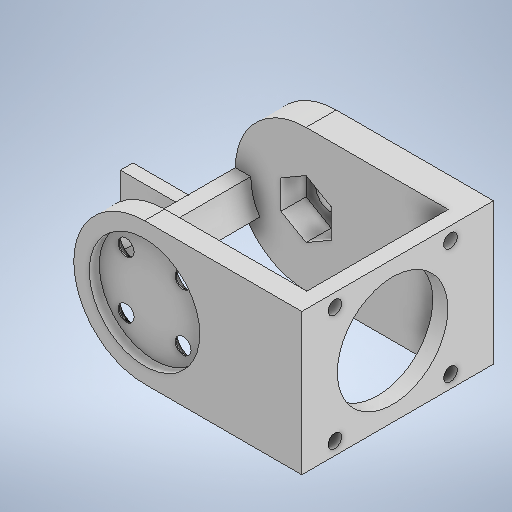
# Autodesk Inventor part: j6 motor mount v2
Saved by Autodesk Inventor 2025 (Build 290162000, 162)
## iProperties
Created: 2025-08-05
Part Number: j6 motor mount v2
Material: 一般
Document SubType Name: Modeling
Designer: gavin
Density: 1 g/cm^3
Appearance: 預設
Author: gavin
## iProperties of the stored document j6 motor mount v2_3D 列印.ipt
Created: 2025-08-05
Part Number: j6 motor mount v2_3D 列印
Material: 一般
Document SubType Name: Modeling
Designer: gavin
Density: 1 g/cm^3
Appearance: 預設
Author: gavin
Autodesk Inventor part; units mm, degrees
ref_plane "YZ Plane" through (0, 0, 0) normal (1, 0, 0) x (0, 1, 0)
ref_plane "XZ Plane" through (0, 0, 0) normal (0, 1, 0) x (-1, 0, 0)
ref_plane "XY Plane" through (0, 0, 0) normal (0, 0, 1) x (1, 0, 0)
sketch "草圖1" plane through (0, 0, 0) normal (1, 0, 0) x (0, 1, 0)
  line L0 (-14.075, 14.075) -> (14.075, 14.075)
  line L1 (14.075, 14.075) -> (14.075, -14.075)
  line L2 (14.075, -14.075) -> (-14.075, -14.075)
  line L3 (-14.075, -14.075) -> (-14.075, 14.075)
  line L4 (-14.075, 14.075) -> (14.075, -14.075) construction
  line L5 (14.075, 14.075) -> (-14.075, -14.075) construction
  line L6 (14.075, 14.075) -> (-14.075, 14.075)
  line L7 (-14.075, 14.075) -> (-14.075, 18.075)
  line L8 (-14.075, 18.075) -> (14.075, 18.075)
  line L9 (14.075, 18.075) -> (14.075, 14.075)
  circle A0 centre (0, 0) radius 11
  line L10 (-11.5, 11.5) -> (11.5, 11.5) construction
  line L11 (11.5, 11.5) -> (11.5, -11.5) construction
  line L12 (11.5, -11.5) -> (-11.5, -11.5) construction
  line L13 (-11.5, -11.5) -> (-11.5, 11.5) construction
  line L14 (-11.5, 11.5) -> (11.5, -11.5) construction
  line L15 (11.5, 11.5) -> (-11.5, -11.5) construction
  circle A1 centre (11.5, 11.5) radius 1.35
  circle A2 centre (-11.5, 11.5) radius 1.35
  circle A3 centre (-11.5, -11.5) radius 1.35
  circle A4 centre (11.5, -11.5) radius 1.35
  line L16 (14.075, -14.075) -> (-14.075, -14.075)
  line L17 (-14.075, -14.075) -> (-14.075, -20.075)
  line L18 (-14.075, -20.075) -> (14.075, -20.075)
  line L19 (14.075, -20.075) -> (14.075, -14.075)
  dimension "d0" = 28.15
  dimension "d1" = 28.15
  dimension "d2" = 4
  dimension "d3" = 22
  dimension "d4" = 23
  dimension "d5" = 23
  dimension "d6" = 2.7
  dimension "d9" = 360
  dimension "d11" = 6
  constraints: 40 end point, 8 parallel, 5 centre point, 4 horizontal, 4 midpoint, 4 perpendicular, 2 coincident, 9 other
  measures "d0" distance of L1.end L2.end
  measures "d1" distance of L0.end L1.end
  measures "d2" distance of L6.end L7.end
  measures "d3" diameter of A0
  measures "d4" distance of L11.end L12.end
  measures "d5" distance of L10.end L11.end
  measures "d6" diameter of A1
  measures "d11" distance of L17.end L16.end
extrude "擠出1" add sketch "草圖1" along normal blind 3
sketch "草圖2" plane through (0, 0, 0) normal (-1, 0, 0) x (0, 0, 1)
  line L0 (18.075, 14.075) -> (18.075, -14.075) projected
  line L1 (-20.075, 14.075) -> (18.075, 14.075) projected
  line L2 (-20.075, -14.075) -> (-20.075, 14.075) projected
  line L3 (18.075, -14.075) -> (-20.075, -14.075) projected
  circle A0 centre (0, 0) radius 11 projected
  circle A1 centre (11.5, 11.5) radius 1.35 projected
  circle A2 centre (11.5, -11.5) radius 1.35 projected
  circle A3 centre (-11.5, -11.5) radius 1.35 projected
  circle A4 centre (-11.5, 11.5) radius 1.35 projected
  line L4 (-14.075, 14.075) -> (-14.075, -14.075)
  line L5 (14.075, 14.075) -> (14.075, -14.075)
  dimension "d14" = 6
  dimension "d15" = 4
  constraints: 4 end point, 4 point on line, 2 vertical
  measures "d14" distance between parallel lines of L2 L4
  measures "d15" distance between parallel lines of L0 L5
extrude "擠出2" add sketch "草圖2" along normal blind 42.375 contours L0 L3 L5 L1 | L4 L3 L2 L1
sketch "草圖3" plane through (3, -14.075, 18.075) normal (0, 0, 1) x (1, 0, 0)
  line L0 (-45.375, 0) -> (0, 0) projected
  line L1 (0, 28.15) -> (0, 0) projected
  line L2 (0, 28.15) -> (-45.375, 28.15) projected
  line L3 (-45.375, 0) -> (-45.375, 28.15) projected
  circle A0 centre (-31.3, 14.075) radius 11
  line L4 (-45.375, 0) -> (-45.375, 28.15) projected
  circle A1 centre (-31.3, 14.075) radius 8 construction
  line L5 (-31.3, 14.075) -> (-23.5218, 21.8532) construction
  line L6 (-31.3, 14.075) -> (-20.3, 14.075) construction
  circle A2 centre (-25.6431, 19.7319) radius 1.6
  circle A3 centre (-36.9569, 19.7319) radius 1.6
  circle A4 centre (-36.9569, 8.4181) radius 1.6
  circle A5 centre (-25.6431, 8.4181) radius 1.6
  point P0 (-3, 14.075)
  dimension "d18" = 22
  dimension "d19" = 16
  dimension "d20" = 45
  dimension "d21" = 3.2
  dimension "d24" = 360
  dimension "d30" = 14.075
  dimension "d31" = 14.075
  constraints: 4 centre point, 4 end point, 1 coincident, 1 equal length, 1 horizontal, 1 horizontal alignment, 1 point on line, 15 other
  measures "d20" angle of L6 L5
  measures "d21" diameter of A2
  measures "d30" distance from line of L2 point (-31.3, 14.075)
  measures "d31" distance from line of L3 point (-31.3, 14.075)
extrude "擠出3" cut sketch "草圖3" against normal up to surface (4 mm away) contours A2 | A3 | A4 | A5
extrude "擠出4" cut sketch "草圖3" against normal blind 2 contours A0
fillet "圓角1" radius 14.075 4 edges at (-42.375, 14.075, 16.075) (-42.375, 14.075, -17.075) (-42.375, -14.075, 16.075) (-42.375, -14.075, -17.075)
sketch "草圖4" plane through (0, -14.075, -14.075) normal (0, 0, 1) x (1, 0, 0)
  circle A0 centre (-28.3, 14.075) radius 11 projected
  line L0 (-28.3, 8.3015) -> (-33.3, 11.1882)
  line L1 (-33.3, 11.1882) -> (-33.3, 16.9618)
  line L2 (-33.3, 16.9618) -> (-28.3, 19.8485)
  line L3 (-28.3, 19.8485) -> (-23.3, 16.9618)
  line L4 (-23.3, 16.9618) -> (-23.3, 11.1882)
  line L5 (-23.3, 11.1882) -> (-28.3, 8.3015)
  point P0 (0, 14.075)
  dimension "d33" = 10
  constraints: 12 end point, 1 coincident, 13 other
  measures "d33" distance between parallel lines of L4 L1
extrude "擠出5" cut sketch "草圖4" against normal blind 5 contours L0 L1 L2 L3 L4 L5
sketch "草圖5" plane through (0, -14.075, -19.075) normal (0, 0, 1) x (1, 0, 0)
  circle A0 centre (-28.3, 14.075) radius 11 projected
  circle A1 centre (-28.3, 14.075) radius 3.1
  point P0 (0, 14.075)
  dimension "d36" = 6.2
  constraints: 1 centre point, 1 coincident
  measures "d36" diameter of A1
extrude "擠出6" cut sketch "草圖5" against normal up to surface (1 mm away) contours A1
sketch "草圖7" plane through (3, 0, 0) normal (1, 0, 0) x (0, 0, -1)
  line L0 (-18.075, 14.075) -> (-18.075, -14.075) projected
  line L1 (-18.075, -14.075) -> (20.075, -14.075) projected
  line L2 (20.075, -14.075) -> (20.075, 14.075) projected
  line L3 (20.075, 14.075) -> (-18.075, 14.075) projected
  circle A0 centre (0, 0) radius 11 projected
  circle A1 centre (-11.5, 11.5) radius 1.35 projected
  circle A2 centre (-11.5, -11.5) radius 1.35 projected
  circle A3 centre (11.5, -11.5) radius 1.35 projected
  circle A4 centre (11.5, 11.5) radius 1.35 projected
  line L4 (-2.75, 14.075) -> (-2.75, 10.6507)
  line L5 (2.75, 14.075) -> (2.75, 10.6507)
  dimension "d44" = 5.5
  dimension "d45" = 2.75
  constraints: 4 end point, 2 point on circle, 2 point on line, 2 vertical
  measures "d44" distance between parallel lines of L5 L4
  measures "d45" distance from line of point (0, 0) L5
sketch "草圖9" plane through (0, -14.075, -14.075) normal (0, 0, 1) x (1, 0, 0)
  line L0 (-47.9197, 8.0745) -> (-57.7197, 8.074) projected
  line L1 (-47.9197, 8.0745) -> (-47.92, 14.1745) projected
  line L2 (-57.72, 14.174) -> (-47.92, 14.1745) projected
  line L3 (-57.7197, 8.074) -> (-57.72, 14.174) projected
  line L4 (-28.3, 19.8485) -> (-23.3, 16.9618) projected
  line L5 (-23.3, 16.9618) -> (-23.3, 11.1882) projected
  line L6 (-23.3, 11.1882) -> (-28.3, 8.3015) projected
  line L7 (-28.3, 8.3015) -> (-33.3, 11.1882) projected
  line L8 (-33.3, 11.1882) -> (-33.3, 16.9618) projected
  line L9 (-33.3, 16.9618) -> (-28.3, 19.8485) projected
  arc A0 (-28.3, 28.15) -> (-28.3, 0) centre (-28.3, 14.075) ccw projected
  line L10 (0, 0) -> (-28.3, 0) projected
  line L11 (0, 28.15) -> (0, 0) projected
  line L12 (0, 28.15) -> (-28.3, 28.15) projected
  line L13 (-41.0318, 8.0745) -> (-36.7075, 8.0745)
  line L14 (-36.7075, 8.0745) -> (-36.7075, 14.1745)
  line L15 (-36.7075, 14.1745) -> (-42.3747, 14.1742)
  circle A1 centre (-28.3, 14.075) radius 3.1 projected
  circle A2 centre (-28.3, 14.075) radius 11
  point P0 (0, 14.075)
  point P1 (-39.8372, 8.0745)
  point P2 (-37.5192, 8.0745)
  point P3 (-39.2996, 14.1744)
  dimension "d54" = 6.1
  dimension "d57" = 22
  constraints: 6 end point, 2 point on circle, 1 centre point, 1 coincident, 1 horizontal, 1 horizontal alignment, 1 parallel, 1 perpendicular, 1 point on line
  measures "d54" distance of L13.end L14.end
  measures "d57" diameter of A2
extrude "擠出10" add sketch "草圖9" along normal up to surface (28.15 mm away) contours L15 A2 L13 A0
ref_plane "工作平面1" through (-55.8797, -6.0007, -3.4552) normal (0, -0.0000388, 1) x (0.0000484, -1, -0.0000388)
sketch "草圖10" plane through (-55.8797, -6.0007, -3.4552) normal (0, -0.0000388, 1) x (0.0000484, -1, -0.0000388)
  ellipse E0 centre (-6.0002, 27.58) end of major axis (-6.0001, 41.655) minor radius 14.075 (-20.0752, 27.5807) -> (8.0748, 27.5793) ccw projected
  line L0 (8.0748, 27.5793) -> (8.0764, 58.8793) projected
  line L1 (-20.0736, 58.8807) -> (8.0764, 58.8793) projected
  line L2 (-20.0736, 58.8807) -> (-20.0752, 27.5807) projected
  ellipse E1 centre (-6.0002, 27.58) end of major axis (-5.9996, 38.58) minor radius 11 projected
  line L3 (-6.0988, 13.5054) -> (-6.0999, 13.5054) projected
  line L4 (-6.0988, 13.5054) -> (-6.0988, 16.5805) projected
  line L5 (0.0012, 18.3605) -> (0.001, 14.8479) projected
  line L6 (-6.0999, 13.5054) -> (-6.0999, 2.5)
  line L7 (-6.0999, 2.5) -> (0.001, 2.5)
  line L8 (0.001, 2.5) -> (0.001, 14.8479)
  line L9 (0, 7.96) -> (0, 0) projected
  line L10 (0, 7.96) -> (-6.1, 7.96) projected
  line L11 (-6.1, 0) -> (-6.1, 7.96) projected
  line L12 (0, 0) -> (-6.1, 0) projected
  point P0 (-5.9981, 55.88)
  point P1 (0.001, 14.8485)
  dimension "d60" = 2.5
  constraints: 6 end point, 2 perpendicular, 1 vertical, 1 other
  measures "d60" distance between parallel lines of L7 L12
extrude "擠出11" add sketch "草圖10" along normal mid plane 2.5 contours E0 L8 L10 L6 | L10 L8 L7 L6
chamfer "倒角1" distance 1.8 angle 45 4 edges at (-35.5569, -5.6569, 14.075) (-35.5569, 5.6569, 14.075) (-24.2431, -5.6569, 14.075) (-24.2431, 5.6569, 14.075)
equation "\"d31\" = d30"
equation "\"d26\" = d19"
equation "\"d45\" = 0.5 * d44"
